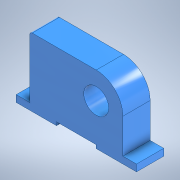
# Autodesk Inventor part: CJ-ACI
Saved by Autodesk Inventor 2022 (Build 260153000, 153)
## iProperties
Created: 2024-10-26
Part Number: CJ-ACI
Material: Ogólny
Document SubType Name: Modeling
Designer: NANOmatic
Density: 1 g/cm^3
Appearance: Cyjan
Author: NANOmatic
Autodesk Inventor part; units mm, degrees
ref_plane "YZ Plane" through (0, 0, 0) normal (1, 0, 0) x (0, 1, 0)
ref_plane "XZ Plane" through (0, 0, 0) normal (0, 1, 0) x (-1, 0, 0)
ref_plane "XY Plane" through (0, 0, 0) normal (0, 0, 1) x (1, 0, 0)
sketch "Szkic1" plane through (0, 0, 0) normal (0, 0, 1) x (1, 0, 0)
  line L0 (53, 0) -> (53, 6)
  line L1 (53, 6) -> (41, 6)
  line L2 (41, 6) -> (41, 36.5)
  line L3 (-53, 0) -> (-53, 6)
  line L4 (-53, 6) -> (-41, 6)
  line L5 (-41, 6) -> (-41, 58)
  line L6 (-39, 60) -> (17.5, 60)
  arc A0 (41, 36.5) -> (17.5, 60) centre (17.5, 36.5) ccw
  circle A1 centre (17.5, 36.5) radius 11
  line L7 (-17.5, 0) -> (-17.5, 3)
  line L8 (-17.5, 3) -> (17.5, 3)
  line L9 (17.5, 3) -> (17.5, 0)
  line L10 (-53, 0) -> (-17.5, 0)
  line L11 (17.5, 0) -> (53, 0)
  line L12 (0, 0) -> (0, 3) construction
  arc A2 (-39, 60) -> (-41, 58) centre (-39, 58) ccw
  point P0 (-41, 60)
  dimension "d0" = 22
  dimension "d1" = 106
  dimension "d3" = 12
  dimension "d4" = 6
  dimension "d5" = 3
  dimension "d6" = 35
  dimension "d7" = 60
  dimension "d10" = 2
  constraints: 26 end point, 9 perpendicular, 6 point on line, 4 point on circle, 4 tangent, 3 centre point, 3 collinear, 2 coincident, 2 horizontal, 2 vertical, 1 midpoint, 1 parallel
  measures "d0" diameter of A1
  measures "d1" distance of L3.start L0.start
  measures "d3" distance of L3.end L4.end
  measures "d4" distance of L3.start L3.end
  measures "d5" distance of L7.start L7.end
  measures "d6" distance of L7.end L8.end
  measures "d7" distance between parallel lines of L10 L6
  measures "d10" radius of A2
extrude "Wyciągnięcie proste1" add sketch "Szkic1" along normal mid plane 24
equation "\"d3\" = 2 * d4"
